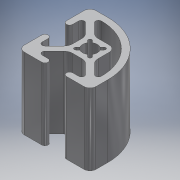
# Autodesk Inventor part: 1012-S
Saved by Autodesk Inventor 2017 SP1 (Build 210196100, 196)
## iProperties
Created: 2016-09-13
Part Number: 1012-S
Material: 6105-T5
Description: 40 S SHORT SINGLE UNIBEARING ASSEMBLY ON 40-4040 X 75mm
Document SubType Name: Modeling
Designer: BRALEF
Density: 1 g/cm^3
Appearance: CLEAR ANODIZED
MATERIAL: 6061-T6
PART PRICE: 44.65
Author: BRALEF
Autodesk Inventor part; units mm, degrees
ref_plane "YZ Plane" through (0, 0, 0) normal (1, 0, 0) x (0, 1, 0)
ref_plane "XZ Plane" through (0, 0, 0) normal (0, 1, 0) x (-1, 0, 0)
ref_plane "XY Plane" through (0, 0, 0) normal (0, 0, 1) x (1, 0, 0)
sketch "Sketch1" plane through (0, 0, 0) normal (0, 1, 0) x (-1, 0, 0)
  arc A0 (-4.5172, 1.6395) -> (-5.4471, 3.8845) centre (-7.6922, 1.6395) ccw
  line L0 (-8.7553, 7.1927) -> (-5.4471, 3.8845)
  arc A1 (-8.7553, 7.1927) -> (-10.4897, 6.4823) centre (-9.4737, 6.4743) ccw
  arc A2 (-10.4897, 6.4823) -> (6.4823, -10.4897) centre (6.35, 6.35) ccw
  arc A3 (6.4823, -10.4897) -> (7.1927, -8.7553) centre (6.4743, -9.4737) ccw
  line L1 (3.8845, -5.4471) -> (7.1927, -8.7553)
  arc A4 (3.8845, -5.4471) -> (1.6395, -4.5172) centre (1.6395, -7.6922) ccw
  line L2 (-2.3074, -4.5172) -> (1.6395, -4.5172)
  arc A5 (-4.5172, -2.3074) -> (-2.3074, -4.5172) centre (-2.3074, -2.3074) ccw
  line L3 (-4.5172, 1.6395) -> (-4.5172, -2.3074)
  arc A6 (-2.2319, 1.3405) -> (-2.2319, -1.3405) centre (0, 0) ccw
  line L4 (-2.8605, -1.9692) -> (-2.2319, -1.3405)
  arc A7 (-2.8605, -1.9692) -> (-1.9692, -2.8605) centre (-2.4696, -2.4696) ccw
  line L5 (-1.3405, -2.2319) -> (-1.9692, -2.8605)
  arc A8 (-1.3405, -2.2319) -> (1.3405, -2.2319) centre (0, 0) ccw
  line L6 (1.9692, -2.8605) -> (1.3405, -2.2319)
  arc A9 (1.9692, -2.8605) -> (2.8605, -1.9692) centre (2.4696, -2.4696) ccw
  line L7 (2.2319, -1.3405) -> (2.8605, -1.9692)
  arc A10 (2.2319, -1.3405) -> (2.2319, 1.3405) centre (0, 0) ccw
  line L8 (2.8605, 1.9692) -> (2.2319, 1.3405)
  arc A11 (2.8605, 1.9692) -> (1.9692, 2.8605) centre (2.4696, 2.4696) ccw
  line L9 (1.3405, 2.2319) -> (1.9692, 2.8605)
  arc A12 (1.3405, 2.2319) -> (-1.3405, 2.2319) centre (0, 0) ccw
  line L10 (-1.9692, 2.8605) -> (-1.3405, 2.2319)
  arc A13 (-1.9692, 2.8605) -> (-2.8605, 1.9692) centre (-2.4696, 2.4696) ccw
  line L11 (-2.2319, 1.3405) -> (-2.8605, 1.9692)
  arc A14 (12.7, -4.3561) -> (10.4902, -4.3561) centre (11.5951, -4.3561) ccw
  line L12 (12.7, -4.3561) -> (12.7, -10.5918)
  arc A15 (10.5918, -12.7) -> (12.7, -10.5918) centre (10.5918, -10.5918) ccw
  line L13 (10.5918, -12.7) -> (6.35, -12.7)
  arc A16 (-12.7, 6.35) -> (6.35, -12.7) centre (6.35, 6.35) ccw
  line L14 (-12.7, 6.35) -> (-12.7, 10.5918)
  arc A17 (-10.5918, 12.7) -> (-12.7, 10.5918) centre (-10.5918, 10.5918) ccw
  line L15 (-10.5918, 12.7) -> (-4.3561, 12.7)
  arc A18 (-4.3561, 10.4902) -> (-4.3561, 12.7) centre (-4.3561, 11.5951) ccw
  line L16 (-4.3561, 10.4902) -> (-6.4749, 10.4902)
  arc A19 (-6.4749, 10.4902) -> (-7.1933, 8.7558) centre (-6.4749, 9.4742) ccw
  line L17 (-7.1933, 8.7558) -> (-3.8846, 5.4471)
  arc A20 (-3.8846, 5.4471) -> (-1.6396, 4.5172) centre (-1.6396, 7.6922) ccw
  line L18 (-1.6396, 4.5172) -> (1.6396, 4.5172)
  arc A21 (1.6396, 4.5172) -> (3.8846, 5.4471) centre (1.6396, 7.6922) ccw
  line L19 (3.8846, 5.4471) -> (7.1933, 8.7558)
  arc A22 (7.1933, 8.7558) -> (6.4749, 10.4902) centre (6.4749, 9.4742) ccw
  line L20 (6.4749, 10.4902) -> (4.3561, 10.4902)
  arc A23 (4.3561, 12.7) -> (4.3561, 10.4902) centre (4.3561, 11.5951) ccw
  line L21 (4.3561, 12.7) -> (10.5918, 12.7)
  arc A24 (12.7, 10.5918) -> (10.5918, 12.7) centre (10.5918, 10.5918) ccw
  line L22 (12.7, 10.5918) -> (12.7, 4.3561)
  arc A25 (10.4902, 4.3561) -> (12.7, 4.3561) centre (11.5951, 4.3561) ccw
  line L23 (10.4902, 4.3561) -> (10.4902, 6.4749)
  arc A26 (10.4902, 6.4749) -> (8.7558, 7.1933) centre (9.4742, 6.4749) ccw
  line L24 (8.7558, 7.1933) -> (5.4471, 3.8846)
  arc A27 (5.4471, 3.8846) -> (4.5172, 1.6396) centre (7.6922, 1.6396) ccw
  line L25 (4.5172, 1.6396) -> (4.5172, -1.6396)
  arc A28 (4.5172, -1.6396) -> (5.4471, -3.8846) centre (7.6922, -1.6396) ccw
  line L26 (5.4471, -3.8846) -> (8.7558, -7.1933)
  arc A29 (8.7558, -7.1933) -> (10.4902, -6.4749) centre (9.4742, -6.4749) ccw
  line L27 (10.4902, -6.4749) -> (10.4902, -4.3561)
  point P0 (0, 0)
  dimension "d0" = 1.1049
  dimension "d1" = 2.1082
  dimension "d2" = 1.016
  dimension "d3" = 3.175
  dimension "d4" = 19.05
  dimension "d5" = 16.8402
  dimension "d6" = 0.635
  dimension "d7" = 2.6035
  dimension "d8" = 2.6035
  dimension "d9" = 2.6035
  dimension "d10" = 2.6035
  dimension "d11" = 2.2098
  dimension "d12" = 45
  dimension "d13" = 45
  dimension "d14" = 45
  dimension "d15" = 45
  dimension "d16" = 45
  dimension "d17" = 45
  dimension "d18" = 90
  dimension "d19" = 45
  dimension "d20" = 90
  dimension "d21" = 90
  dimension "d22" = 90
  dimension "d23" = 8.1828
  dimension "d24" = 17.2172
  dimension "d25" = 25.4
  dimension "d26" = 25.4
  dimension "d27" = 17.2172
  dimension "d28" = 8.1828
  dimension "d29" = 2.2096
  dimension "d30" = 1.7351
  dimension "d31" = 0.4746
  dimension "d32" = 1.7352
  dimension "d33" = 0.4746
  dimension "d34" = 2.2097
  dimension "d35" = 12.7
  dimension "d36" = 12.7
  dimension "d37" = 10.4902
  dimension "d38" = 12.7
  dimension "d39" = 1.1048
  dimension "d40" = 1.1048
  dimension "d41" = 1.1049
  dimension "d42" = 0.6303
  dimension "d43" = 0.6303
  dimension "d44" = 0.6303
  dimension "d45" = 0.6303
  dimension "d46" = 10.4902
  dimension "d47" = 1.1049
  dimension "d48" = 12.7
  dimension "d49" = 17.0561
  dimension "d50" = 8.3439
  dimension "d51" = 8.3439
  dimension "d52" = 9.8395
  dimension "d53" = 9.8395
  dimension "d54" = 10.2304
  dimension "d55" = 10.2304
  dimension "d56" = 10.4681
  dimension "d57" = 10.4681
  dimension "d58" = 14.6692
  dimension "d59" = 14.6692
  dimension "d60" = 15.1696
  dimension "d61" = 15.1696
  dimension "d62" = 17.0561
  constraints: 60 point on circle, 56 end point, 42 tangent, 30 centre point, 16 equal radius, 14 parallel, 1 horizontal, 1 perpendicular, 1 vertical
  measures "d0" radius of A25
  measures "d1" radius of A24
  measures "d2" radius of A26
  measures "d3" radius of A27
  measures "d4" radius of A16
  measures "d5" radius of A2
  measures "d6" radius of A11
  measures "d7" radius of A8
  measures "d8" radius of A10
  measures "d9" radius of A12
  measures "d10" radius of A6
  measures "d11" radius of A5
  measures "d12" angle of L22 L24
  measures "d13" angle of L22 L26
  measures "d14" angle of L22 L8
  measures "d15" angle of L22 L10
  measures "d16" angle of L22 L11
  measures "d17" angle of L22 L4
  measures "d18" angle of L22 L16
  measures "d19" angle of L22 L0
  measures "d20" angle of L15 L22
  measures "d21" angle of L12 L13
  measures "d22" angle of L13 L27
  measures "d23" distance between parallel lines of L22 L25
  measures "d24" distance between parallel lines of L3 L22
  measures "d25" distance between parallel lines of L14 L22
  measures "d26" distance between parallel lines of L13 L21
  measures "d27" distance between parallel lines of L13 L18
  measures "d28" distance between parallel lines of L2 L13
  measures "d29" distance between parallel lines of L24 L19
  measures "d30" distance between parallel lines of L9 L24
  measures "d31" distance between parallel lines of L5 L24
  measures "d32" distance between parallel lines of L7 L1
  measures "d33" distance between parallel lines of L6 L1
  measures "d34" distance between parallel lines of L1 L17
  measures "d35" distance from line of point (0, 0) L22
  measures "d36" distance from line of point (0, 0) L12
  measures "d37" distance from line of point (0, 0) L27
  measures "d38" distance from line of point (0, 0) L13
  measures "d39" distance from line of point (0, 0) L24
  measures "d40" distance from line of point (0, 0) L26
  measures "d41" distance from line of point (0, 0) L1
  measures "d42" distance from line of point (0, 0) L8
  measures "d43" distance from line of point (0, 0) L10
  measures "d44" distance from line of point (0, 0) L11
  measures "d45" distance from line of point (0, 0) L4
  measures "d46" distance from line of point (0, 0) L16
  measures "d47" distance from line of point (0, 0) L0
  measures "d48" distance from line of point (0, 0) L15
  measures "d49" distance from line of L22.end L13
  measures "d50" distance from line of L12.start L13
  measures "d51" distance from line of L21.start L22
  measures "d52" distance from line of L8.start L22
  measures "d53" distance from line of L7.end L22
  measures "d54" distance from line of A11.centre L22
  measures "d55" distance from line of A9.centre L22
  measures "d56" distance from line of L8.end L22
  measures "d57" distance from line of L7.start L22
  measures "d58" distance from line of L10.start L22
  measures "d59" distance from line of L5.end L22
  measures "d60" distance from line of A13.centre L22
  measures "d61" distance from line of A7.centre L22
  measures "d62" distance from line of L15.end L22
extrude "Extrusion1" add sketch "Sketch1" along normal mid plane 25.4
body "Solid1"
